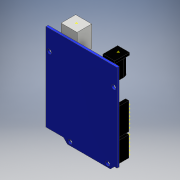
# Autodesk Inventor part: ArduinoUno
Saved by Autodesk Inventor 2016 (Build 200138000, 138)
## iProperties
Created: 2015-09-20
Part Number: ArduinoUno
Material: GFRP
Document SubType Name: Modeling
Designer: Artur
Density: 1.75 g/cm^3
Appearance: Smooth - Light Gray
Mass: 16.8005 g
Surface Area: 132.112 cm^2
Volume: 9.60028 cm^3
Author: Artur
Autodesk Inventor part; units mm, degrees
(part 1 of 3)
ref_plane "YZ Plane" through (0, 0, 0) normal (1, 0, 0) x (0, 1, 0)
ref_plane "XZ Plane" through (0, 0, 0) normal (0, 1, 0) x (-1, 0, 0)
sketch "Sketch1" plane through (0, 0, 0) normal (0, 1, 0) x (-1, 0, 0)
  line L0 (0, 0) -> (-53, 0)
  line L1 (-53, 0) -> (-53, -65)
  line L2 (-53, -65) -> (-51, -65)
  line L3 (-48, -68) -> (-16, -68)
  line L4 (-48, -68) -> (-51, -65)
  line L5 (0, -65) -> (-13, -65)
  circle A0 centre (-2.5, -15) radius 1.6
  circle A1 centre (-50.5, -13.9) radius 1.6
  circle A2 centre (-46, -65.5) radius 1.6
  circle A3 centre (-18, -65.5) radius 1.6
  line L6 (0, 0) -> (0, -93.7538) construction
  line L7 (-16, -68) -> (-13, -65)
  line L8 (0, -65) -> (0, 0)
  dimension "d0" = 53
  dimension "d1" = 65
  dimension "d2" = 2
  dimension "d3" = 32
  dimension "d4" = 68
  dimension "d5" = 5
  dimension "d6" = 13
  dimension "d7" = 3.2
  dimension "d9" = 15
  dimension "d10" = 3.2
  dimension "d11" = 1.1
  dimension "d12" = 2.5
  dimension "d13" = 3.2
  dimension "d14" = 3.2
  dimension "d15" = 7
  dimension "d16" = 65.5
  dimension "d17" = 35
  dimension "d18" = 65.5
  dimension "d20" = 2.5
  constraints: 18 end point, 4 centre point, 4 horizontal, 1 coincident, 1 collinear, 1 perpendicular, 1 point on line, 1 vertical
  measures "d0" distance of L0.start L0.end
  measures "d1" distance of L0.end L1.end
  measures "d2" distance of L1.end L2.end
  measures "d3" distance of L3.start L3.end
  measures "d4" distance between parallel lines of L0 L3
  measures "d5" distance from line of L1 L3.start
  measures "d6" distance of L5.start L5.end
  measures "d7" diameter of A0
  measures "d9" distance from line of L0 A0.centre
  measures "d10" diameter of A1
  measures "d11" vertical distance of A0.centre A1.centre
  measures "d12" distance from line of L1 A1.centre
  measures "d13" diameter of A2
  measures "d14" diameter of A3
  measures "d15" distance from line of L1 A2.centre
  measures "d16" distance from line of L0 A2.centre
  measures "d17" distance from line of L1 A3.centre
  measures "d18" distance from line of L0 A3.centre
  measures "d20" distance from line of L8 A0.centre
extrude "board" add sketch "Sketch1" against normal blind 1.6
sketch "Sketch2" plane through (0, 0, 0) normal (0, 1, 0) x (1, 0, 0)
  line L0 (9.6, 9.8) -> (9.6, -6.2)
  line L1 (9.6, -6.2) -> (21.6, -6.2)
  line L2 (21.6, -6.2) -> (21.6, 9.8)
  line L3 (21.6, 9.8) -> (9.6, 9.8)
  line L4 (0, 65) -> (0, 0) projected
  line L5 (0, 0) -> (53, 0) projected
  dimension "d23" = 16
  dimension "d24" = 12
  dimension "d25" = 9.6
  dimension "d26" = 9.8
  constraints: 8 end point, 3 perpendicular, 1 vertical
  measures "d23" distance of L0.start L0.end
  measures "d24" distance of L0.end L1.end
  measures "d25" distance between parallel lines of L4 L0
  measures "d26" distance between parallel lines of L5 L3
extrude "serialPort" add sketch "Sketch2" along normal blind 10.9 separate body
sketch "Sketch3" plane through (0, 0, 0) normal (0, 1, 0) x (1, 0, 0)
  line L0 (40.8, 12.2) -> (40.8, -1.8)
  line L1 (40.8, -1.8) -> (49.7, -1.8)
  line L2 (49.7, -1.8) -> (49.7, 12.2)
  line L3 (49.7, 12.2) -> (40.8, 12.2)
  line L4 (0, 0) -> (53, 0) projected
  line L5 (53, 0) -> (53, 65) projected
  dimension "d29" = 14
  dimension "d30" = 8.9
  dimension "d31" = 1.8
  dimension "d32" = 3.3
  constraints: 8 end point, 3 perpendicular, 1 vertical
  measures "d29" distance of L0.start L0.end
  measures "d30" distance of L0.end L1.end
  measures "d31" distance between parallel lines of L1 L4
  measures "d32" distance between parallel lines of L5 L2
extrude "powerPort" add sketch "Sketch3" along normal blind 11 separate body
sketch "Sketch4" plane through (0, 11, 0) normal (0, 1, 0) x (1, 0, 0)
  line L0 (0, 0) -> (53, 0) projected
split body "powerPortSplit" sketch "Sketch4" result two bodies bodies 3 curves L0 first body at (49.2, 3.6667, -4.0667)
fillet "powerPortFillet" radius 4.45 2 edges at (40.8, 11, -6.1) (49.7, 11, -6.1)
sketch "Sketch5" plane through (0, 0, 0) normal (0, 1, 0) x (1, 0, 0)
  line L0 (1.25, 43.5) -> (3.75, 43.5)
  line L1 (3.75, 43.5) -> (3.75, 18.5)
  line L2 (3.75, 18.5) -> (1.25, 18.5)
  line L3 (1.25, 18.5) -> (1.25, 43.5)
  line L4 (0, 65) -> (0, 0) projected
  line L5 (0, 0) -> (53, 0) projected
  line L6 (1.25, 64) -> (3.75, 64)
  line L7 (3.75, 64) -> (3.75, 44)
  line L8 (3.75, 44) -> (1.25, 44)
  line L9 (1.25, 44) -> (1.25, 64)
  line L10 (13, 65) -> (0, 65) projected
  line L11 (51.75, 64) -> (49.25, 64)
  line L12 (49.25, 64) -> (49.25, 49)
  line L13 (49.25, 49) -> (51.75, 49)
  line L14 (51.75, 49) -> (51.75, 64)
  line L15 (51.75, 47) -> (49.25, 47)
  line L16 (49.25, 27) -> (51.75, 27)
  line L17 (51.75, 47) -> (51.75, 27)
  line L18 (49.25, 47) -> (49.25, 27)
  point P0 (53, 65)
  dimension "d36" = 2.5
  dimension "d37" = 25
  dimension "d38" = 1.25
  dimension "d39" = 43.5
  dimension "d40" = 20
  dimension "d41" = 2.5
  dimension "d42" = 1
  dimension "d43" = 1.25
  dimension "d44" = 2.5
  dimension "d45" = 2.5
  dimension "d46" = 20
  dimension "d47" = 15
  dimension "d48" = 1.25
  dimension "d49" = 1
  dimension "d50" = 2
  constraints: 32 end point, 7 parallel, 4 horizontal, 3 perpendicular, 2 vertical, 1 point on line
  measures "d36" distance of L1.end L2.end
  measures "d37" distance of L0.end L1.end
  measures "d38" distance between parallel lines of L4 L3
  measures "d39" distance between parallel lines of L5 L0
  measures "d40" distance of L6.end L7.end
  measures "d41" distance of L7.end L8.end
  measures "d42" distance from line of L10 L6.start
  measures "d43" distance between parallel lines of L4 L9
  measures "d44" distance of L11.start L11.end
  measures "d45" distance of L15.start L15.end
  measures "d46" distance of L16.end L15.start
  measures "d47" distance of L13.end L11.start
  measures "d48" horizontal distance of point (53, 65) L11.start
  measures "d49" vertical distance of L11.start point (53, 65)
  measures "d50" distance of L15.start L13.end
extrude "pinsBase" add sketch "Sketch5" along normal blind 8.5 separate body
sketch "sketch6" plane through (0, 8.5, 0) normal (0, 1, 0) x (1, 0, 0)
  line L0 (1.5, 63.75) -> (3.5, 63.75)
  line L1 (3.5, 63.75) -> (3.5, 61.75)
  line L2 (3.5, 61.75) -> (1.5, 61.75)
  line L3 (1.5, 61.75) -> (1.5, 63.75)
  line L4 (3.75, 64) -> (1.25, 64) construction
  line L5 (1.25, 64) -> (1.25, 44) construction
  line L6 (1.5, 61.25) -> (3.5, 61.25)
  line L7 (3.5, 61.25) -> (3.5, 59.25)
  line L8 (3.5, 59.25) -> (1.5, 59.25)
  line L9 (1.5, 59.25) -> (1.5, 61.25)
  line L10 (1.5, 58.75) -> (3.5, 58.75)
  line L11 (3.5, 58.75) -> (3.5, 56.75)
  line L12 (3.5, 56.75) -> (1.5, 56.75)
  line L13 (1.5, 56.75) -> (1.5, 58.75)
  line L14 (1.5, 56.25) -> (3.5, 56.25)
  line L15 (3.5, 56.25) -> (3.5, 54.25)
  line L16 (3.5, 54.25) -> (1.5, 54.25)
  line L17 (1.5, 54.25) -> (1.5, 56.25)
  line L18 (1.5, 53.75) -> (3.5, 53.75)
  line L19 (3.5, 53.75) -> (3.5, 51.75)
  line L20 (3.5, 51.75) -> (1.5, 51.75)
  line L21 (1.5, 51.75) -> (1.5, 53.75)
  line L22 (1.5, 51.25) -> (3.5, 51.25)
  line L23 (3.5, 51.25) -> (3.5, 49.25)
  line L24 (3.5, 49.25) -> (1.5, 49.25)
  line L25 (1.5, 49.25) -> (1.5, 51.25)
  line L26 (1.5, 48.75) -> (3.5, 48.75)
  line L27 (3.5, 48.75) -> (3.5, 46.75)
  line L28 (3.5, 46.75) -> (1.5, 46.75)
  line L29 (1.5, 46.75) -> (1.5, 48.75)
  line L30 (1.5, 46.25) -> (3.5, 46.25)
  line L31 (3.5, 46.25) -> (3.5, 44.25)
  line L32 (3.5, 44.25) -> (1.5, 44.25)
  line L33 (1.5, 44.25) -> (1.5, 46.25)
  line L34 (3.75, 43.5) -> (1.25, 43.5) construction
  line L35 (1.25, 43.5) -> (1.25, 18.5) construction
  line L36 (1.5, 43.25) -> (3.5, 43.25)
  line L37 (3.5, 43.25) -> (3.5, 41.25)
  line L38 (3.5, 41.25) -> (1.5, 41.25)
  line L39 (1.5, 41.25) -> (1.5, 43.25)
  line L40 (1.5, 40.75) -> (3.5, 40.75)
  line L41 (3.5, 40.75) -> (3.5, 38.75)
  line L42 (3.5, 38.75) -> (1.5, 38.75)
  line L43 (1.5, 38.75) -> (1.5, 40.75)
  line L44 (1.5, 38.25) -> (3.5, 38.25)
  line L45 (3.5, 38.25) -> (3.5, 36.25)
  line L46 (3.5, 36.25) -> (1.5, 36.25)
  line L47 (1.5, 36.25) -> (1.5, 38.25)
  line L48 (1.5, 35.75) -> (3.5, 35.75)
  line L49 (3.5, 35.75) -> (3.5, 33.75)
  line L50 (3.5, 33.75) -> (1.5, 33.75)
  line L51 (1.5, 33.75) -> (1.5, 35.75)
  line L52 (1.5, 33.25) -> (3.5, 33.25)
  line L53 (3.5, 33.25) -> (3.5, 31.25)
  line L54 (3.5, 31.25) -> (1.5, 31.25)
  line L55 (1.5, 31.25) -> (1.5, 33.25)
  line L56 (1.5, 30.75) -> (3.5, 30.75)
  line L57 (3.5, 30.75) -> (3.5, 28.75)
  line L58 (3.5, 28.75) -> (1.5, 28.75)
  line L59 (1.5, 28.75) -> (1.5, 30.75)
  line L60 (1.5, 28.25) -> (3.5, 28.25)
  line L61 (3.5, 28.25) -> (3.5, 26.25)
  line L62 (3.5, 26.25) -> (1.5, 26.25)
  line L63 (1.5, 26.25) -> (1.5, 28.25)
  line L64 (1.5, 25.75) -> (3.5, 25.75)
  line L65 (3.5, 25.75) -> (3.5, 23.75)
  line L66 (3.5, 23.75) -> (1.5, 23.75)
  line L67 (1.5, 23.75) -> (1.5, 25.75)
  line L68 (1.5, 23.25) -> (3.5, 23.25)
  line L69 (3.5, 23.25) -> (3.5, 21.25)
  line L70 (3.5, 21.25) -> (1.5, 21.25)
  line L71 (1.5, 21.25) -> (1.5, 23.25)
  line L72 (1.5, 20.75) -> (3.5, 20.75)
  line L73 (3.5, 20.75) -> (3.5, 18.75)
  line L74 (3.5, 18.75) -> (1.5, 18.75)
  line L75 (1.5, 18.75) -> (1.5, 20.75)
  line L76 (49.5, 63.75) -> (51.5, 63.75)
  line L77 (51.5, 63.75) -> (51.5, 61.75)
  line L78 (51.5, 61.75) -> (49.5, 61.75)
  line L79 (49.5, 61.75) -> (49.5, 63.75)
  line L80 (49.5, 46.75) -> (51.5, 46.75)
  line L81 (51.5, 46.75) -> (51.5, 44.75)
  line L82 (51.5, 44.75) -> (49.5, 44.75)
  line L83 (49.5, 44.75) -> (49.5, 46.75)
  line L84 (51.75, 64) -> (49.25, 64) construction
  line L85 (49.25, 64) -> (49.25, 49) construction
  line L86 (51.75, 47) -> (49.25, 47) construction
  line L87 (49.25, 47) -> (49.25, 27) construction
  line L88 (51.5, 59.25) -> (49.5, 59.25)
  line L89 (49.5, 59.25) -> (49.5, 61.25)
  line L90 (49.5, 61.25) -> (51.5, 61.25)
  line L91 (51.5, 61.25) -> (51.5, 59.25)
  line L92 (51.5, 56.75) -> (49.5, 56.75)
  line L93 (49.5, 56.75) -> (49.5, 58.75)
  line L94 (49.5, 58.75) -> (51.5, 58.75)
  line L95 (51.5, 58.75) -> (51.5, 56.75)
  line L96 (51.5, 54.25) -> (49.5, 54.25)
  line L97 (49.5, 54.25) -> (49.5, 56.25)
  line L98 (49.5, 56.25) -> (51.5, 56.25)
  line L99 (51.5, 56.25) -> (51.5, 54.25)
  line L100 (51.5, 51.75) -> (49.5, 51.75)
  line L101 (49.5, 51.75) -> (49.5, 53.75)
  line L102 (49.5, 53.75) -> (51.5, 53.75)
  line L103 (51.5, 53.75) -> (51.5, 51.75)
  line L104 (51.5, 49.25) -> (49.5, 49.25)
  line L105 (49.5, 49.25) -> (49.5, 51.25)
  line L106 (49.5, 51.25) -> (51.5, 51.25)
  line L107 (51.5, 51.25) -> (51.5, 49.25)
  line L108 (49.5, 44.25) -> (51.5, 44.25)
  line L109 (49.5, 42.25) -> (49.5, 44.25)
  line L110 (51.5, 42.25) -> (49.5, 42.25)
  line L111 (51.5, 44.25) -> (51.5, 42.25)
  line L112 (49.5, 41.75) -> (51.5, 41.75)
  line L113 (49.5, 39.75) -> (49.5, 41.75)
  line L114 (51.5, 39.75) -> (49.5, 39.75)
  line L115 (51.5, 41.75) -> (51.5, 39.75)
  line L116 (49.5, 39.25) -> (51.5, 39.25)
  line L117 (49.5, 37.25) -> (49.5, 39.25)
  line L118 (51.5, 37.25) -> (49.5, 37.25)
  line L119 (51.5, 39.25) -> (51.5, 37.25)
  line L120 (49.5, 36.75) -> (51.5, 36.75)
  line L121 (49.5, 34.75) -> (49.5, 36.75)
  line L122 (51.5, 34.75) -> (49.5, 34.75)
  line L123 (51.5, 36.75) -> (51.5, 34.75)
  line L124 (49.5, 34.25) -> (51.5, 34.25)
  line L125 (49.5, 32.25) -> (49.5, 34.25)
  line L126 (51.5, 32.25) -> (49.5, 32.25)
  line L127 (51.5, 34.25) -> (51.5, 32.25)
  line L128 (49.5, 31.75) -> (51.5, 31.75)
  line L129 (49.5, 29.75) -> (49.5, 31.75)
  line L130 (51.5, 29.75) -> (49.5, 29.75)
  line L131 (51.5, 31.75) -> (51.5, 29.75)
  line L132 (49.5, 29.25) -> (51.5, 29.25)
  line L133 (49.5, 27.25) -> (49.5, 29.25)
  line L134 (51.5, 27.25) -> (49.5, 27.25)
  line L135 (51.5, 29.25) -> (51.5, 27.25)
  point P0 (0, 0)
  dimension "d53" = 2
  dimension "d54" = 2
  dimension "d55" = 0.25
  dimension "d56" = 0.25
  dimension "d61" = 2.5
  dimension "d70" = 2
  dimension "d71" = 2
  dimension "d72" = 0.25
  dimension "d73" = 0.25
  dimension "d76" = 2.5
  dimension "d89" = 2
  dimension "d90" = 2
  dimension "d99" = 2
  dimension "d100" = 2
  dimension "d101" = 0.25
  dimension "d102" = 0.25
  dimension "d103" = 0.25
  dimension "d104" = 0.25
  dimension "d107" = 2.5
  dimension "d114" = 2.5
  constraints: 256 end point, 8 parallel, 4 horizontal, 4 perpendicular, 4 vertical, 224 other
  measures "d53" distance of L1.end L2.end
  measures "d54" distance of L0.end L1.end
  measures "d55" distance from line of L4 L0.end
  measures "d56" distance from line of L5 L0.start
  measures "d61" distance of L0.start L6.start
  measures "d70" distance of L37.end L38.end
  measures "d71" distance of L37.start L37.end
  measures "d72" distance between parallel lines of L34 L36
  measures "d73" distance between parallel lines of L35 L39
  measures "d76" distance of L37.start L40.end
  measures "d89" distance of L78.start L78.end
  measures "d90" distance of L76.end L78.start
  measures "d99" distance of L82.start L82.end
  measures "d100" distance of L80.end L82.start
  measures "d101" distance between parallel lines of L86 L80
  measures "d102" distance between parallel lines of L87 L83
  measures "d103" distance between parallel lines of L84 L76
  measures "d104" distance between parallel lines of L85 L79
  measures "d107" distance of L78.end L88.end
  measures "d114" distance of L80.end L108.end
extrude "pinHoles" cut sketch "sketch6" against normal up to next bodies 6
sketch "pinLabelsSketch" plane through (0, 0, 0) normal (0, 1, 0) x (1, 0, 0)
  line L0 (10.8569, 44) -> (4, 44) construction
  line L1 (4, 44) -> (4, 64) construction
  line L2 (4, 64) -> (10.8569, 64) construction
  line L3 (10.8569, 64) -> (10.8569, 44) construction
  line L4 (3.5, 61.75) -> (1.5, 61.75) construction
  line L5 (3.75, 44) -> (3.75, 64) construction
  line L6 (1.25, 44) -> (3.75, 44) construction
  line L7 (3.75, 64) -> (1.25, 64) construction
  line L8 (10.2543, 23.75) -> (4, 23.75) construction
  line L9 (4, 23.75) -> (4, 43.5) construction
  line L10 (4, 43.5) -> (10.2543, 43.5) construction
  line L11 (10.2543, 43.5) -> (10.2543, 23.75) construction
  line L12 (3.75, 18.5) -> (3.75, 43.5) construction
  line L13 (1.25, 18.5) -> (3.75, 18.5) construction
  line L14 (3.75, 43.5) -> (1.25, 43.5) construction
  line L15 (3.5, 23.75) -> (1.5, 23.75) construction
  line L16 (49, 49) -> (44.6855, 49) construction
  line L17 (44.6855, 49) -> (44.6855, 64) construction
  line L18 (44.6855, 64) -> (49, 64) construction
  line L19 (49, 64) -> (49, 49) construction
  line L20 (49.25, 64) -> (49.25, 49) construction
  line L21 (51.75, 64) -> (49.25, 64) construction
  line L22 (49.25, 49) -> (51.75, 49) projected
  line L23 (49, 47) -> (49, 29.75) construction
  line L24 (49, 29.75) -> (42.6731, 29.75) construction
  line L25 (42.6731, 29.75) -> (42.6731, 47) construction
  line L26 (42.6731, 47) -> (49, 47) construction
  line L27 (49.25, 47) -> (49.25, 27) construction
  line L28 (49.25, 27) -> (51.75, 27) projected
  line L29 (51.75, 47) -> (49.25, 47) construction
  line L30 (51.5, 29.75) -> (49.5, 29.75) construction
  line L31 (48.3254, 31.6408) -> (48.9064, 31.6408)
  line L32 (48.9064, 31.6408) -> (48.9064, 31.4876)
  line L33 (48.9064, 31.4876) -> (48.7156, 31.4876)
  line L34 (48.7156, 31.4876) -> (48.7156, 30.294)
  line L35 (48.7156, 30.294) -> (48.9064, 30.294)
  line L36 (48.9064, 30.294) -> (48.9064, 30.1408)
  line L37 (48.9064, 30.1408) -> (48.3254, 30.1408)
  line L38 (48.3254, 30.1408) -> (48.3254, 30.294)
  line L39 (48.3254, 30.294) -> (48.5162, 30.294)
  line L40 (48.5162, 30.294) -> (48.5162, 31.4876)
  line L41 (48.5162, 31.4876) -> (48.3254, 31.4876)
  line L42 (48.3254, 31.4876) -> (48.3254, 31.6408)
  spline S0 degree 2 poles (47.0174, 30.3122) (46.9323, 30.4119) (46.8375, 30.7036) (46.8375, 30.8908) knots 0 0 0 1 2 2 2
  spline S1 degree 2 poles (46.8375, 30.8908) (46.8375, 31.0731) (46.9299, 31.3685) (47.0174, 31.4682) knots 0 0 0 1 2 2 2
  spline S2 degree 2 poles (47.0174, 31.4682) (47.1098, 31.5727) (47.3541, 31.6724) (47.5012, 31.6724) knots 0 0 0 1 2 2 2
  spline S3 degree 2 poles (47.5012, 31.6724) (47.6532, 31.6724) (47.8963, 31.5691) (47.985, 31.4682) knots 0 0 0 1 2 2 2
  spline S4 degree 2 poles (47.985, 31.4682) (48.0713, 31.3685) (48.1637, 31.0756) (48.1637, 30.8908) knots 0 0 0 1 2 2 2
  spline S5 degree 2 poles (48.1637, 30.8908) (48.1637, 30.7024) (48.0701, 30.4155) (47.9838, 30.3122) knots 0 0 0 1 2 2 2
  spline S6 degree 2 poles (47.9838, 30.3122) (47.8963, 30.2125) (47.6519, 30.1092) (47.5012, 30.1092) knots 0 0 0 1 2 2 2
  spline S7 degree 2 poles (47.5012, 30.1092) (47.3481, 30.1092) (47.1025, 30.2162) (47.0174, 30.3122) knots 0 0 0 1 2 2 2
  spline S8 degree 2 poles (47.0454, 30.8908) (47.0454, 30.7425) (47.1098, 30.5128) (47.1682, 30.4374) knots 0 0 0 1 2 2 2
  spline S9 degree 2 poles (47.1682, 30.4374) (47.2277, 30.3596) (47.3955, 30.2818) (47.5, 30.2818) knots 0 0 0 1 2 2 2
  spline S10 degree 2 poles (47.5, 30.2818) (47.6082, 30.2818) (47.7711, 30.3572) (47.8331, 30.4374) knots 0 0 0 1 2 2 2
  spline S11 degree 2 poles (47.8331, 30.4374) (47.8926, 30.514) (47.9558, 30.7449) (47.9558, 30.8908) knots 0 0 0 1 2 2 2
  spline S12 degree 2 poles (47.9558, 30.8908) (47.9558, 31.1862) (47.7079, 31.4998) (47.5, 31.4998) knots 0 0 0 1 2 2 2
  spline S13 degree 2 poles (47.5, 31.4998) (47.2921, 31.4998) (47.0454, 31.1862) (47.0454, 30.8908) knots 0 0 0 1 2 2 2
  line L43 (45.4579, 31.6408) -> (45.7168, 31.6408)
  line L44 (45.7168, 31.6408) -> (46.1908, 31.044)
  line L45 (46.1908, 31.044) -> (46.4194, 31.044)
  line L46 (46.4194, 31.044) -> (46.4194, 31.6408)
  line L47 (46.4194, 31.6408) -> (46.6187, 31.6408)
  line L48 (46.6187, 31.6408) -> (46.6187, 30.1408)
  line L49 (46.6187, 30.1408) -> (46.2322, 30.1408)
  spline S14 degree 2 poles (46.2322, 30.1408) (46.1033, 30.1408) (45.9295, 30.1688) (45.8505, 30.2198) knots 0 0 0 1 2 2 2
  spline S15 degree 2 poles (45.8505, 30.2198) (45.7715, 30.2709) (45.6803, 30.4301) (45.6803, 30.548) knots 0 0 0 1 2 2 2
  spline S16 degree 2 poles (45.6803, 30.548) (45.6803, 30.7121) (45.8481, 30.9346) (45.9915, 30.988) knots 0 0 0 1 2 2 2
  line L50 (45.9915, 30.988) -> (45.4579, 31.6408)
  spline S17 degree 2 poles (45.8882, 30.5638) (45.8882, 30.4982) (45.9344, 30.3973) (45.983, 30.3645) knots 0 0 0 1 2 2 2
  spline S18 degree 2 poles (45.983, 30.3645) (46.0255, 30.3365) (46.1386, 30.3134) (46.2212, 30.3134) knots 0 0 0 1 2 2 2
  line L51 (46.2212, 30.3134) -> (46.4194, 30.3134)
  line L52 (46.4194, 30.3134) -> (46.4194, 30.8774)
  line L53 (46.4194, 30.8774) -> (46.2443, 30.8774)
  spline S19 degree 2 poles (46.2443, 30.8774) (46.158, 30.8774) (46.0207, 30.847) (45.9733, 30.7996) knots 0 0 0 1 2 2 2
  spline S20 degree 2 poles (45.9733, 30.7996) (45.9295, 30.7583) (45.8882, 30.6416) (45.8882, 30.5638) knots 0 0 0 1 2 2 2
  line L54 (45.3387, 31.6408) -> (45.3387, 30.1408)
  line L55 (45.3387, 30.1408) -> (44.4003, 30.1408)
  line L56 (44.4003, 30.1408) -> (44.4003, 30.3183)
  line L57 (44.4003, 30.3183) -> (45.1394, 30.3183)
  line L58 (45.1394, 30.3183) -> (45.1394, 30.7291)
  line L59 (45.1394, 30.7291) -> (44.4502, 30.7291)
  line L60 (44.4502, 30.7291) -> (44.4502, 30.9066)
  line L61 (44.4502, 30.9066) -> (45.1394, 30.9066)
  line L62 (45.1394, 30.9066) -> (45.1394, 31.4633)
  line L63 (45.1394, 31.4633) -> (44.4003, 31.4633)
  line L64 (44.4003, 31.4633) -> (44.4003, 31.6408)
  line L65 (44.4003, 31.6408) -> (45.3387, 31.6408)
  line L66 (43.2844, 30.3183) -> (43.9822, 30.3183)
  line L67 (43.9822, 30.3183) -> (43.9822, 30.7413)
  line L68 (43.9822, 30.7413) -> (43.3136, 30.7413)
  line L69 (43.3136, 30.7413) -> (43.3136, 30.9188)
  line L70 (43.3136, 30.9188) -> (43.9822, 30.9188)
  line L71 (43.9822, 30.9188) -> (43.9822, 31.6408)
  line L72 (43.9822, 31.6408) -> (44.1815, 31.6408)
  line L73 (44.1815, 31.6408) -> (44.1815, 30.1408)
  line L74 (44.1815, 30.1408) -> (43.2844, 30.1408)
  line L75 (43.2844, 30.1408) -> (43.2844, 30.3183)
  line L76 (47.6872, 34.1408) -> (47.9461, 34.1408)
  line L77 (47.9461, 34.1408) -> (48.4202, 33.544)
  line L78 (48.4202, 33.544) -> (48.6487, 33.544)
  line L79 (48.6487, 33.544) -> (48.6487, 34.1408)
  line L80 (48.6487, 34.1408) -> (48.8481, 34.1408)
  line L81 (48.8481, 34.1408) -> (48.8481, 32.6408)
  line L82 (48.8481, 32.6408) -> (48.4615, 32.6408)
  spline S21 degree 2 poles (48.4615, 32.6408) (48.3327, 32.6408) (48.1588, 32.6688) (48.0798, 32.7198) knots 0 0 0 1 2 2 2
  spline S22 degree 2 poles (48.0798, 32.7198) (48.0008, 32.7709) (47.9096, 32.9301) (47.9096, 33.048) knots 0 0 0 1 2 2 2
  spline S23 degree 2 poles (47.9096, 33.048) (47.9096, 33.2121) (48.0774, 33.4346) (48.2208, 33.488) knots 0 0 0 1 2 2 2
  line L83 (48.2208, 33.488) -> (47.6872, 34.1408)
  spline S24 degree 2 poles (48.1175, 33.0638) (48.1175, 32.9982) (48.1637, 32.8973) (48.2123, 32.8645) knots 0 0 0 1 2 2 2
  spline S25 degree 2 poles (48.2123, 32.8645) (48.2549, 32.8365) (48.3679, 32.8134) (48.4506, 32.8134) knots 0 0 0 1 2 2 2
  line L84 (48.4506, 32.8134) -> (48.6487, 32.8134)
  line L85 (48.6487, 32.8134) -> (48.6487, 33.3774)
  line L86 (48.6487, 33.3774) -> (48.4737, 33.3774)
  spline S26 degree 2 poles (48.4737, 33.3774) (48.3874, 33.3774) (48.25, 33.347) (48.2026, 33.2996) knots 0 0 0 1 2 2 2
  spline S27 degree 2 poles (48.2026, 33.2996) (48.1588, 33.2583) (48.1175, 33.1416) (48.1175, 33.0638) knots 0 0 0 1 2 2 2
  line L87 (47.5681, 34.1408) -> (47.5681, 32.6408)
  line L88 (47.5681, 32.6408) -> (46.6297, 32.6408)
  line L89 (46.6297, 32.6408) -> (46.6297, 32.8183)
  line L90 (46.6297, 32.8183) -> (47.3687, 32.8183)
  line L91 (47.3687, 32.8183) -> (47.3687, 33.2291)
  line L92 (47.3687, 33.2291) -> (46.6795, 33.2291)
  line L93 (46.6795, 33.2291) -> (46.6795, 33.4066)
  line L94 (46.6795, 33.4066) -> (47.3687, 33.4066)
  line L95 (47.3687, 33.4066) -> (47.3687, 33.9633)
  line L96 (47.3687, 33.9633) -> (46.6297, 33.9633)
  line L97 (46.6297, 33.9633) -> (46.6297, 34.1408)
  line L98 (46.6297, 34.1408) -> (47.5681, 34.1408)
  spline S28 degree 2 poles (45.9927, 34.1675) (46.1556, 34.1675) (46.3841, 34.0995) (46.485, 34.0509) knots 0 0 0 1 2 2 2
  line L99 (46.485, 34.0509) -> (46.485, 33.8004)
  line L100 (46.485, 33.8004) -> (46.4704, 33.8004)
  spline S29 degree 2 poles (46.4704, 33.8004) (46.372, 33.8928) (46.1228, 33.9949) (46.0073, 33.9949) knots 0 0 0 1 2 2 2
  spline S30 degree 2 poles (46.0073, 33.9949) (45.842, 33.9949) (45.673, 33.8576) (45.673, 33.7445) knots 0 0 0 1 2 2 2
  spline S31 degree 2 poles (45.673, 33.7445) (45.673, 33.6546) (45.7618, 33.5427) (45.8578, 33.5148) knots 0 0 0 1 2 2 2
  spline S32 degree 2 poles (45.8578, 33.5148) (45.9271, 33.4953) (46.0425, 33.4686) (46.1288, 33.4467) knots 0 0 0 1 2 2 2
  spline S33 degree 2 poles (46.1288, 33.4467) (46.2066, 33.4261) (46.3294, 33.3641) (46.3768, 33.3142) knots 0 0 0 1 2 2 2
  spline S34 degree 2 poles (46.3768, 33.3142) (46.423, 33.2644) (46.4741, 33.1307) (46.4741, 33.0432) knots 0 0 0 1 2 2 2
  spline S35 degree 2 poles (46.4741, 33.0432) (46.4741, 32.8608) (46.1896, 32.6141) (45.9696, 32.6141) knots 0 0 0 1 2 2 2
  spline S36 degree 2 poles (45.9696, 32.6141) (45.8432, 32.6141) (45.6195, 32.6639) (45.5235, 32.7113) knots 0 0 0 1 2 2 2
  line L101 (45.5235, 32.7113) -> (45.5235, 32.9496)
  line L102 (45.5235, 32.9496) -> (45.5381, 32.9496)
  spline S37 degree 2 poles (45.5381, 32.9496) (45.6098, 32.8839) (45.8335, 32.7867) (45.9562, 32.7867) knots 0 0 0 1 2 2 2
  spline S38 degree 2 poles (45.9562, 32.7867) (46.0948, 32.7867) (46.2662, 32.9167) (46.2662, 33.0225) knots 0 0 0 1 2 2 2
  spline S39 degree 2 poles (46.2662, 33.0225) (46.2662, 33.1173) (46.1653, 33.2303) (46.0705, 33.2559) knots 0 0 0 1 2 2 2
  spline S40 degree 2 poles (46.0705, 33.2559) (46.0073, 33.2729) (45.8237, 33.3167) (45.763, 33.3349) knots 0 0 0 1 2 2 2
  spline S41 degree 2 poles (45.763, 33.3349) (45.6086, 33.3823) (45.4652, 33.5731) (45.4652, 33.7129) knots 0 0 0 1 2 2 2
  spline S42 degree 2 poles (45.4652, 33.7129) (45.4652, 33.8017) (45.5369, 33.9718) (45.6013, 34.0314) knots 0 0 0 1 2 2 2
  spline S43 degree 2 poles (45.6013, 34.0314) (45.673, 34.097) (45.8553, 34.1675) (45.9927, 34.1675) knots 0 0 0 1 2 2 2
  line L103 (45.2622, 34.1408) -> (45.2622, 32.6408)
  line L104 (45.2622, 32.6408) -> (44.3237, 32.6408)
  line L105 (44.3237, 32.6408) -> (44.3237, 32.8183)
  line L106 (44.3237, 32.8183) -> (45.0628, 32.8183)
  line L107 (45.0628, 32.8183) -> (45.0628, 33.2291)
  line L108 (45.0628, 33.2291) -> (44.3736, 33.2291)
  line L109 (44.3736, 33.2291) -> (44.3736, 33.4066)
  line L110 (44.3736, 33.4066) -> (45.0628, 33.4066)
  line L111 (45.0628, 33.4066) -> (45.0628, 33.9633)
  line L112 (45.0628, 33.9633) -> (44.3237, 33.9633)
  line L113 (44.3237, 33.9633) -> (44.3237, 34.1408)
  line L114 (44.3237, 34.1408) -> (45.2622, 34.1408)
  line L115 (43.7549, 34.1408) -> (43.7549, 32.8183)
  line L116 (43.7549, 32.8183) -> (44.2581, 32.8183)
  line L117 (44.2581, 32.8183) -> (44.2581, 32.6408)
  line L118 (44.2581, 32.6408) -> (43.0523, 32.6408)
  line L119 (43.0523, 32.6408) -> (43.0523, 32.8183)
  line L120 (43.0523, 32.8183) -> (43.5555, 32.8183)
  line L121 (43.5555, 32.8183) -> (43.5555, 34.1408)
  line L122 (43.5555, 34.1408) -> (43.7549, 34.1408)
  spline S44 degree 2 poles (48.4858, 35.283) (48.5405, 35.283) (48.6487, 35.3098) (48.701, 35.3304) knots 0 0 0 1 2 2 2
  spline S45 degree 2 poles (48.701, 35.3304) (48.7496, 35.3511) (48.8213, 35.3949) (48.8493, 35.4143) knots 0 0 0 1 2 2 2
  line L123 (48.8493, 35.4143) -> (48.8614, 35.4143)
  line L124 (48.8614, 35.4143) -> (48.8614, 35.2016)
  spline S46 degree 2 poles (48.8614, 35.2016) (48.7958, 35.1663) (48.5709, 35.1092) (48.47, 35.1092) knots 0 0 0 1 2 2 2
  spline S47 degree 2 poles (48.47, 35.1092) (48.3679, 35.1092) (48.216, 35.1505) (48.154, 35.1943) knots 0 0 0 1 2 2 2
  spline S48 degree 2 poles (48.154, 35.1943) (48.0883, 35.2417) (48.0203, 35.3791) (48.0203, 35.4714) knots 0 0 0 1 2 2 2
  spline S49 degree 2 poles (48.0203, 35.4714) (48.0203, 35.5954) (48.1831, 35.7826) (48.2974, 35.8069) knots 0 0 0 1 2 2 2
  line L125 (48.2974, 35.8069) -> (48.2974, 35.8215)
  spline S50 degree 2 poles (48.2974, 35.8215) (48.25, 35.8312) (48.1418, 35.875) (48.0956, 35.9188) knots 0 0 0 1 2 2 2
  spline S51 degree 2 poles (48.0956, 35.9188) (48.0494, 35.9613) (47.9911, 36.0974) (47.9911, 36.1959) knots 0 0 0 1 2 2 2
  spline S52 degree 2 poles (47.9911, 36.1959) (47.9911, 36.2968) (48.0604, 36.4682) (48.1236, 36.5338) knots 0 0 0 1 2 2 2
  spline S53 degree 2 poles (48.1236, 36.5338) (48.1892, 36.6019) (48.3752, 36.6724) (48.4931, 36.6724) knots 0 0 0 1 2 2 2
  spline S54 degree 2 poles (48.4931, 36.6724) (48.6062, 36.6724) (48.8274, 36.6177) (48.9028, 36.58) knots 0 0 0 1 2 2 2
  line L126 (48.9028, 36.58) -> (48.9028, 36.3673)
  line L127 (48.9028, 36.3673) -> (48.8882, 36.3673)
  spline S55 degree 2 poles (48.8882, 36.3673) (48.825, 36.4135) (48.611, 36.4986) (48.5053, 36.4986) knots 0 0 0 1 2 2 2
  spline S56 degree 2 poles (48.5053, 36.4986) (48.4433, 36.4986) (48.3193, 36.4597) (48.278, 36.4147) knots 0 0 0 1 2 2 2
  spline S57 degree 2 poles (48.278, 36.4147) (48.2378, 36.3697) (48.1953, 36.2628) (48.1953, 36.1813) knots 0 0 0 1 2 2 2
  spline S58 degree 2 poles (48.1953, 36.1813) (48.1953, 36.0999) (48.2427, 35.9941) (48.2853, 35.9637) knots 0 0 0 1 2 2 2
  spline S59 degree 2 poles (48.2853, 35.9637) (48.3278, 35.9333) (48.4433, 35.9103) (48.5113, 35.9103) knots 0 0 0 1 2 2 2
  line L128 (48.5113, 35.9103) -> (48.5964, 35.9103)
  line L129 (48.5964, 35.9103) -> (48.5964, 35.7437)
  line L130 (48.5964, 35.7437) -> (48.5296, 35.7437)
  spline S60 degree 2 poles (48.5296, 35.7437) (48.3947, 35.7437) (48.2245, 35.6149) (48.2245, 35.4921) knots 0 0 0 1 2 2 2
  spline S61 degree 2 poles (48.2245, 35.4921) (48.2245, 35.435) (48.2682, 35.3535) (48.3035, 35.3292) knots 0 0 0 1 2 2 2
  spline S62 degree 2 poles (48.3035, 35.3292) (48.3412, 35.3037) (48.4335, 35.283) (48.4858, 35.283) knots 0 0 0 1 2 2 2
  line L131 (47.4429, 36.6408) -> (47.6835, 36.6408)
  line L132 (47.6835, 36.6408) -> (47.6835, 36.3539)
  line L133 (47.6835, 36.3539) -> (47.4429, 36.3539)
  line L134 (47.4429, 36.3539) -> (47.4429, 36.6408)
  spline S63 degree 2 poles (46.7354, 35.283) (46.7901, 35.283) (46.8983, 35.3098) (46.9506, 35.3304) knots 0 0 0 1 2 2 2
  spline S64 degree 2 poles (46.9506, 35.3304) (46.9992, 35.3511) (47.0709, 35.3949) (47.0989, 35.4143) knots 0 0 0 1 2 2 2
  line L135 (47.0989, 35.4143) -> (47.111, 35.4143)
  line L136 (47.111, 35.4143) -> (47.111, 35.2016)
  spline S65 degree 2 poles (47.111, 35.2016) (47.0454, 35.1663) (46.8205, 35.1092) (46.7196, 35.1092) knots 0 0 0 1 2 2 2
  spline S66 degree 2 poles (46.7196, 35.1092) (46.6175, 35.1092) (46.4656, 35.1505) (46.4036, 35.1943) knots 0 0 0 1 2 2 2
  spline S67 degree 2 poles (46.4036, 35.1943) (46.3379, 35.2417) (46.2699, 35.3791) (46.2699, 35.4714) knots 0 0 0 1 2 2 2
  spline S68 degree 2 poles (46.2699, 35.4714) (46.2699, 35.5954) (46.4327, 35.7826) (46.547, 35.8069) knots 0 0 0 1 2 2 2
  line L137 (46.547, 35.8069) -> (46.547, 35.8215)
  spline S69 degree 2 poles (46.547, 35.8215) (46.4996, 35.8312) (46.3914, 35.875) (46.3452, 35.9188) knots 0 0 0 1 2 2 2
  spline S70 degree 2 poles (46.3452, 35.9188) (46.299, 35.9613) (46.2407, 36.0974) (46.2407, 36.1959) knots 0 0 0 1 2 2 2
  spline S71 degree 2 poles (46.2407, 36.1959) (46.2407, 36.2968) (46.31, 36.4682) (46.3732, 36.5338) knots 0 0 0 1 2 2 2
  spline S72 degree 2 poles (46.3732, 36.5338) (46.4388, 36.6019) (46.6248, 36.6724) (46.7427, 36.6724) knots 0 0 0 1 2 2 2
  spline S73 degree 2 poles (46.7427, 36.6724) (46.8558, 36.6724) (47.077, 36.6177) (47.1524, 36.58) knots 0 0 0 1 2 2 2
  line L138 (47.1524, 36.58) -> (47.1524, 36.3673)
  line L139 (47.1524, 36.3673) -> (47.1378, 36.3673)
  spline S74 degree 2 poles (47.1378, 36.3673) (47.0746, 36.4135) (46.8606, 36.4986) (46.7549, 36.4986) knots 0 0 0 1 2 2 2
  spline S75 degree 2 poles (46.7549, 36.4986) (46.6929, 36.4986) (46.5689, 36.4597) (46.5276, 36.4147) knots 0 0 0 1 2 2 2
  spline S76 degree 2 poles (46.5276, 36.4147) (46.4874, 36.3697) (46.4449, 36.2628) (46.4449, 36.1813) knots 0 0 0 1 2 2 2
  spline S77 degree 2 poles (46.4449, 36.1813) (46.4449, 36.0999) (46.4923, 35.9941) (46.5348, 35.9637) knots 0 0 0 1 2 2 2
  spline S78 degree 2 poles (46.5348, 35.9637) (46.5774, 35.9333) (46.6929, 35.9103) (46.7609, 35.9103) knots 0 0 0 1 2 2 2
  line L140 (46.7609, 35.9103) -> (46.846, 35.9103)
  line L141 (46.846, 35.9103) -> (46.846, 35.7437)
  line L142 (46.846, 35.7437) -> (46.7792, 35.7437)
  spline S79 degree 2 poles (46.7792, 35.7437) (46.6442, 35.7437) (46.4741, 35.6149) (46.4741, 35.4921) knots 0 0 0 1 2 2 2
  spline S80 degree 2 poles (46.4741, 35.4921) (46.4741, 35.435) (46.5178, 35.3535) (46.5531, 35.3292) knots 0 0 0 1 2 2 2
  spline S81 degree 2 poles (46.5531, 35.3292) (46.5908, 35.3037) (46.6831, 35.283) (46.7354, 35.283) knots 0 0 0 1 2 2 2
  line L143 (44.8841, 35.1408) -> (45.4007, 36.6408)
  line L144 (45.4007, 36.6408) -> (45.6159, 36.6408)
  line L145 (45.6159, 36.6408) -> (46.1325, 35.1408)
  line L146 (46.1325, 35.1408) -> (45.9186, 35.1408)
  line L147 (45.9186, 35.1408) -> (45.5028, 36.3868)
  line L148 (45.5028, 36.3868) -> (45.0871, 35.1408)
  line L149 (45.0871, 35.1408) -> (44.8841, 35.1408)
  spline S82 degree 2 poles (47.9814, 38.6643) (47.9814, 38.7725) (48.0506, 38.9573) (48.1139, 39.0253) knots 0 0 0 1 2 2 2
  spline S83 degree 2 poles (48.1139, 39.0253) (48.1771, 39.0934) (48.3655, 39.1724) (48.4822, 39.1724) knots 0 0 0 1 2 2 2
  spline S84 degree 2 poles (48.4822, 39.1724) (48.5891, 39.1724) (48.7982, 39.125) (48.8748, 39.0873) knots 0 0 0 1 2 2 2
  line L150 (48.8748, 39.0873) -> (48.8748, 38.8746)
  line L151 (48.8748, 38.8746) -> (48.8602, 38.8746)
  spline S85 degree 2 poles (48.8602, 38.8746) (48.8371, 38.8916) (48.7508, 38.9354) (48.6985, 38.9548) knots 0 0 0 1 2 2 2
  spline S86 degree 2 poles (48.6985, 38.9548) (48.639, 38.9755) (48.5405, 38.9986) (48.4785, 38.9986) knots 0 0 0 1 2 2 2
  spline S87 degree 2 poles (48.4785, 38.9986) (48.4177, 38.9986) (48.3035, 38.9548) (48.2622, 38.9074) knots 0 0 0 1 2 2 2
  spline S88 degree 2 poles (48.2622, 38.9074) (48.2245, 38.8624) (48.1856, 38.7433) (48.1856, 38.6631) knots 0 0 0 1 2 2 2
  spline S89 degree 2 poles (48.1856, 38.6631) (48.1856, 38.5829) (48.2293, 38.4808) (48.2707, 38.4467) knots 0 0 0 1 2 2 2
  spline S90 degree 2 poles (48.2707, 38.4467) (48.3132, 38.409) (48.4396, 38.3774) (48.5162, 38.3774) knots 0 0 0 1 2 2 2
  spline S91 degree 2 poles (48.5162, 38.3774) (48.5989, 38.3774) (48.763, 38.403) (48.8128, 38.4139) knots 0 0 0 1 2 2 2
  line L152 (48.8128, 38.4139) -> (48.8128, 37.6408)
  line L153 (48.8128, 37.6408) -> (47.9899, 37.6408)
  line L154 (47.9899, 37.6408) -> (47.9899, 37.8171)
  line L155 (47.9899, 37.8171) -> (48.6195, 37.8171)
  line L156 (48.6195, 37.8171) -> (48.6195, 38.217)
  spline S92 degree 2 poles (48.6195, 38.217) (48.5831, 38.2121) (48.5126, 38.2085) (48.4834, 38.2085) knots 0 0 0 1 2 2 2
  spline S93 degree 2 poles (48.4834, 38.2085) (48.3679, 38.2085) (48.2087, 38.2462) (48.1357, 38.3021) knots 0 0 0 1 2 2 2
  spline S94 degree 2 poles (48.1357, 38.3021) (48.0616, 38.358) (47.9814, 38.5282) (47.9814, 38.6643) knots 0 0 0 1 2 2 2
  line L157 (46.6345, 37.6408) -> (47.1511, 39.1408)
  line L158 (47.1511, 39.1408) -> (47.3663, 39.1408)
  line L159 (47.3663, 39.1408) -> (47.8829, 37.6408)
  line L160 (47.8829, 37.6408) -> (47.669, 37.6408)
  line L161 (47.669, 37.6408) -> (47.2532, 38.8868)
  line L162 (47.2532, 38.8868) -> (46.8375, 37.6408)
  line L163 (46.8375, 37.6408) -> (46.6345, 37.6408)
  spline S95 degree 2 poles (48.2196, 41.67) (48.3788, 41.67) (48.6426, 41.5727) (48.7374, 41.4743) knots 0 0 0 1 2 2 2
  spline S96 degree 2 poles (48.7374, 41.4743) (48.8323, 41.3746) (48.9331, 41.0804) (48.9331, 40.8896) knots 0 0 0 1 2 2 2
  spline S97 degree 2 poles (48.9331, 40.8896) (48.9331, 40.7085) (48.831, 40.4216) (48.7362, 40.3195) knots 0 0 0 1 2 2 2
  spline S98 degree 2 poles (48.7362, 40.3195) (48.6451, 40.221) (48.3776, 40.1141) (48.2184, 40.1141) knots 0 0 0 1 2 2 2
  spline S99 degree 2 poles (48.2184, 40.1141) (48.1418, 40.1141) (48.0032, 40.1359) (47.94, 40.1554) knots 0 0 0 1 2 2 2
  spline S100 degree 2 poles (47.94, 40.1554) (47.889, 40.17) (47.765, 40.2235) (47.7273, 40.2429) knots 0 0 0 1 2 2 2
  line L164 (47.7273, 40.2429) -> (47.7273, 40.4836)
  line L165 (47.7273, 40.4836) -> (47.7443, 40.4836)
  spline S101 degree 2 poles (47.7443, 40.4836) (47.782, 40.4508) (47.861, 40.3912) (47.934, 40.3572) knots 0 0 0 1 2 2 2
  spline S102 degree 2 poles (47.934, 40.3572) (47.9947, 40.3268) (48.1515, 40.2867) (48.2415, 40.2867) knots 0 0 0 1 2 2 2
  spline S103 degree 2 poles (48.2415, 40.2867) (48.4579, 40.2867) (48.7253, 40.6124) (48.7253, 40.8835) knots 0 0 0 1 2 2 2
  spline S104 degree 2 poles (48.7253, 40.8835) (48.7253, 41.0342) (48.6548, 41.2603) (48.5879, 41.3381) knots 0 0 0 1 2 2 2
  spline S105 degree 2 poles (48.5879, 41.3381) (48.5235, 41.4159) (48.3412, 41.4974) (48.2269, 41.4974) knots 0 0 0 1 2 2 2
  spline S106 degree 2 poles (48.2269, 41.4974) (48.143, 41.4974) (47.9753, 41.4731) (47.9182, 41.4487) knots 0 0 0 1 2 2 2
  line L166 (47.9182, 41.4487) -> (47.9182, 41.061)
  line L167 (47.9182, 41.061) -> (48.2658, 41.061)
  line L168 (48.2658, 41.061) -> (48.2658, 40.8859)
  line L169 (48.2658, 40.8859) -> (47.7212, 40.8859)
  line L170 (47.7212, 40.8859) -> (47.7212, 41.5411)
  spline S107 degree 2 poles (47.7212, 41.5411) (47.7589, 41.5581) (47.8878, 41.6104) (47.9425, 41.6262) knots 0 0 0 1 2 2 2
  spline S108 degree 2 poles (47.9425, 41.6262) (48.0166, 41.6481) (48.1357, 41.67) (48.2196, 41.67) knots 0 0 0 1 2 2 2
  line L171 (46.3975, 41.6408) -> (46.6212, 41.6408)
  line L172 (46.6212, 41.6408) -> (47.2848, 40.3474)
  line L173 (47.2848, 40.3474) -> (47.2848, 41.6408)
  line L174 (47.2848, 41.6408) -> (47.4708, 41.6408)
  line L175 (47.4708, 41.6408) -> (47.4708, 40.1408)
  line L176 (47.4708, 40.1408) -> (47.1876, 40.1408)
  line L177 (47.1876, 40.1408) -> (46.5835, 41.3284)
  line L178 (46.5835, 41.3284) -> (46.5835, 40.1408)
  line L179 (46.5835, 40.1408) -> (46.3975, 40.1408)
  line L180 (46.3975, 40.1408) -> (46.3975, 41.6408)
  spline S109 degree 2 poles (44.9109, 40.892) (44.9109, 41.0974) (45.0774, 41.4281) (45.2172, 41.5205) knots 0 0 0 1 2 2 2
  spline S110 degree 2 poles (45.2172, 41.5205) (45.3314, 41.5922) (45.566, 41.6408) (45.7484, 41.6408) knots 0 0 0 1 2 2 2
  line L181 (45.7484, 41.6408) -> (46.0936, 41.6408)
  line L182 (46.0936, 41.6408) -> (46.0936, 40.1408)
  line L183 (46.0936, 40.1408) -> (45.752, 40.1408)
  spline S111 degree 2 poles (45.752, 40.1408) (45.5405, 40.1408) (45.2998, 40.204) (45.2147, 40.2599) knots 0 0 0 1 2 2 2
  spline S112 degree 2 poles (45.2147, 40.2599) (45.0701, 40.356) (44.9109, 40.6732) (44.9109, 40.892) knots 0 0 0 1 2 2 2
  spline S113 degree 2 poles (45.1187, 40.8896) (45.1187, 40.717) (45.233, 40.4726) (45.346, 40.4034) knots 0 0 0 1 2 2 2
  spline S114 degree 2 poles (45.346, 40.4034) (45.4263, 40.356) (45.6074, 40.3134) (45.7423, 40.3134) knots 0 0 0 1 2 2 2
  line L184 (45.7423, 40.3134) -> (45.8942, 40.3134)
  line L185 (45.8942, 40.3134) -> (45.8942, 41.4682)
  line L186 (45.8942, 41.4682) -> (45.7423, 41.4682)
  spline S115 degree 2 poles (45.7423, 41.4682) (45.6098, 41.4682) (45.4092, 41.4256) (45.3278, 41.3685) knots 0 0 0 1 2 2 2
  spline S116 degree 2 poles (45.3278, 41.3685) (45.2233, 41.298) (45.1187, 41.0646) (45.1187, 40.8896) knots 0 0 0 1 2 2 2
  spline S117 degree 2 poles (48.2196, 44.17) (48.3788, 44.17) (48.6426, 44.0727) (48.7374, 43.9743) knots 0 0 0 1 2 2 2
  spline S118 degree 2 poles (48.7374, 43.9743) (48.8323, 43.8746) (48.9331, 43.5804) (48.9331, 43.3896) knots 0 0 0 1 2 2 2
  spline S119 degree 2 poles (48.9331, 43.3896) (48.9331, 43.2085) (48.831, 42.9216) (48.7362, 42.8195) knots 0 0 0 1 2 2 2
  spline S120 degree 2 poles (48.7362, 42.8195) (48.6451, 42.721) (48.3776, 42.6141) (48.2184, 42.6141) knots 0 0 0 1 2 2 2
  spline S121 degree 2 poles (48.2184, 42.6141) (48.1418, 42.6141) (48.0032, 42.6359) (47.94, 42.6554) knots 0 0 0 1 2 2 2
  spline S122 degree 2 poles (47.94, 42.6554) (47.889, 42.67) (47.765, 42.7235) (47.7273, 42.7429) knots 0 0 0 1 2 2 2
  line L187 (47.7273, 42.7429) -> (47.7273, 42.9836)
  line L188 (47.7273, 42.9836) -> (47.7443, 42.9836)
  spline S123 degree 2 poles (47.7443, 42.9836) (47.782, 42.9508) (47.861, 42.8912) (47.934, 42.8572) knots 0 0 0 1 2 2 2
  spline S124 degree 2 poles (47.934, 42.8572) (47.9947, 42.8268) (48.1515, 42.7867) (48.2415, 42.7867) knots 0 0 0 1 2 2 2
  spline S125 degree 2 poles (48.2415, 42.7867) (48.4579, 42.7867) (48.7253, 43.1124) (48.7253, 43.3835) knots 0 0 0 1 2 2 2
  spline S126 degree 2 poles (48.7253, 43.3835) (48.7253, 43.5342) (48.6548, 43.7603) (48.5879, 43.8381) knots 0 0 0 1 2 2 2
  spline S127 degree 2 poles (48.5879, 43.8381) (48.5235, 43.9159) (48.3412, 43.9974) (48.2269, 43.9974) knots 0 0 0 1 2 2 2
  spline S128 degree 2 poles (48.2269, 43.9974) (48.143, 43.9974) (47.9753, 43.9731) (47.9182, 43.9487) knots 0 0 0 1 2 2 2
  line L189 (47.9182, 43.9487) -> (47.9182, 43.561)
  line L190 (47.9182, 43.561) -> (48.2658, 43.561)
  line L191 (48.2658, 43.561) -> (48.2658, 43.3859)
  line L192 (48.2658, 43.3859) -> (47.7212, 43.3859)
  line L193 (47.7212, 43.3859) -> (47.7212, 44.0411)
  spline S129 degree 2 poles (47.7212, 44.0411) (47.7589, 44.0581) (47.8878, 44.1104) (47.9425, 44.1262) knots 0 0 0 1 2 2 2
  spline S130 degree 2 poles (47.9425, 44.1262) (48.0166, 44.1481) (48.1357, 44.17) (48.2196, 44.17) knots 0 0 0 1 2 2 2
  line L194 (46.3975, 44.1408) -> (46.6212, 44.1408)
  line L195 (46.6212, 44.1408) -> (47.2848, 42.8474)
  line L196 (47.2848, 42.8474) -> (47.2848, 44.1408)
  line L197 (47.2848, 44.1408) -> (47.4708, 44.1408)
  line L198 (47.4708, 44.1408) -> (47.4708, 42.6408)
  line L199 (47.4708, 42.6408) -> (47.1876, 42.6408)
  line L200 (47.1876, 42.6408) -> (46.5835, 43.8284)
  line L201 (46.5835, 43.8284) -> (46.5835, 42.6408)
  line L202 (46.5835, 42.6408) -> (46.3975, 42.6408)
  line L203 (46.3975, 42.6408) -> (46.3975, 44.1408)
  spline S131 degree 2 poles (44.9109, 43.392) (44.9109, 43.5974) (45.0774, 43.9281) (45.2172, 44.0205) knots 0 0 0 1 2 2 2
  spline S132 degree 2 poles (45.2172, 44.0205) (45.3314, 44.0922) (45.566, 44.1408) (45.7484, 44.1408) knots 0 0 0 1 2 2 2
  line L204 (45.7484, 44.1408) -> (46.0936, 44.1408)
  line L205 (46.0936, 44.1408) -> (46.0936, 42.6408)
  line L206 (46.0936, 42.6408) -> (45.752, 42.6408)
  spline S133 degree 2 poles (45.752, 42.6408) (45.5405, 42.6408) (45.2998, 42.704) (45.2147, 42.7599) knots 0 0 0 1 2 2 2
  spline S134 degree 2 poles (45.2147, 42.7599) (45.0701, 42.856) (44.9109, 43.1732) (44.9109, 43.392) knots 0 0 0 1 2 2 2
  spline S135 degree 2 poles (45.1187, 43.3896) (45.1187, 43.217) (45.233, 42.9726) (45.346, 42.9034) knots 0 0 0 1 2 2 2
  spline S136 degree 2 poles (45.346, 42.9034) (45.4263, 42.856) (45.6074, 42.8134) (45.7423, 42.8134) knots 0 0 0 1 2 2 2
  line L207 (45.7423, 42.8134) -> (45.8942, 42.8134)
  line L208 (45.8942, 42.8134) -> (45.8942, 43.9682)
  line L209 (45.8942, 43.9682) -> (45.7423, 43.9682)
  spline S137 degree 2 poles (45.7423, 43.9682) (45.6098, 43.9682) (45.4092, 43.9256) (45.3278, 43.8685) knots 0 0 0 1 2 2 2
  spline S138 degree 2 poles (45.3278, 43.8685) (45.2233, 43.798) (45.1187, 43.5646) (45.1187, 43.3896) knots 0 0 0 1 2 2 2
  line L210 (47.7601, 45.1408) -> (48.2767, 46.6408)
  line L211 (48.2767, 46.6408) -> (48.4919, 46.6408)
  line L212 (48.4919, 46.6408) -> (49.0085, 45.1408)
  line L213 (49.0085, 45.1408) -> (48.7946, 45.1408)
  line L214 (48.7946, 45.1408) -> (48.3788, 46.3868)
  line L215 (48.3788, 46.3868) -> (47.9631, 45.1408)
  line L216 (47.9631, 45.1408) -> (47.7601, 45.1408)
  line L217 (47.438, 46.6408) -> (47.6276, 46.6408)
  line L218 (47.6276, 46.6408) -> (47.6276, 45.5152)
  line L219 (47.6276, 45.5152) -> (47.438, 45.5152)
  line L220 (47.438, 45.5152) -> (47.438, 46.6408)
  line L221 (47.4246, 45.328) -> (47.6398, 45.328)
  line L222 (47.6398, 45.328) -> (47.6398, 45.1311)
  line L223 (47.6398, 45.1311) -> (47.4246, 45.1311)
  line L224 (47.4246, 45.1311) -> (47.4246, 45.328)
  line L225 (46.2759, 46.6408) -> (46.4656, 46.6408)
  line L226 (46.4656, 46.6408) -> (46.4656, 45.999)
  spline S139 degree 2 poles (46.4656, 45.999) (46.4656, 45.9212) (46.4801, 45.7875) (46.502, 45.7474) knots 0 0 0 1 2 2 2
  spline S140 degree 2 poles (46.502, 45.7474) (46.5251, 45.7048) (46.6078, 45.6635) (46.6783, 45.6635) knots 0 0 0 1 2 2 2
  spline S141 degree 2 poles (46.6783, 45.6635) (46.7488, 45.6635) (46.8983, 45.7389) (46.97, 45.7996) knots 0 0 0 1 2 2 2
  line L227 (46.97, 45.7996) -> (46.97, 46.6408)
  line L228 (46.97, 46.6408) -> (47.1596, 46.6408)
  line L229 (47.1596, 46.6408) -> (47.1596, 45.5152)
  line L230 (47.1596, 45.5152) -> (46.97, 45.5152)
  line L231 (46.97, 45.5152) -> (46.97, 45.6404)
  spline S142 degree 2 poles (46.97, 45.6404) (46.8849, 45.5638) (46.7208, 45.4836) (46.6284, 45.4836) knots 0 0 0 1 2 2 2
  spline S143 degree 2 poles (46.6284, 45.4836) (46.4631, 45.4836) (46.2759, 45.7024) (46.2759, 45.9103) knots 0 0 0 1 2 2 2
  line L232 (46.2759, 45.9103) -> (46.2759, 46.6408)
  line L233 (49.0097, 50.9994) -> (48.5041, 49.4994)
  line L234 (48.5041, 49.4994) -> (48.2585, 49.4994)
  line L235 (48.2585, 49.4994) -> (47.7528, 50.9994)
  line L236 (47.7528, 50.9994) -> (47.9631, 50.9994)
  line L237 (47.9631, 50.9994) -> (48.0993, 50.58)
  line L238 (48.0993, 50.58) -> (48.6718, 50.58)
  line L239 (48.6718, 50.58) -> (48.8079, 50.9994)
  line L240 (48.8079, 50.9994) -> (49.0097, 50.9994)
  line L241 (48.154, 50.4098) -> (48.3861, 49.7036)
  line L242 (48.3861, 49.7036) -> (48.6171, 50.4098)
  line L243 (48.6171, 50.4098) -> (48.154, 50.4098)
  spline S144 degree 2 poles (46.7196, 50.2494) (46.7196, 50.653) (46.9542, 51.031) (47.1985, 51.031) knots 0 0 0 1 2 2 2
  spline S145 degree 2 poles (47.1985, 51.031) (47.4465, 51.031) (47.6787, 50.6457) (47.6787, 50.2506) knots 0 0 0 1 2 2 2
  spline S146 degree 2 poles (47.6787, 50.2506) (47.6787, 49.8446) (47.4441, 49.469) (47.1985, 49.469) knots 0 0 0 1 2 2 2
  spline S147 degree 2 poles (47.1985, 49.469) (46.9518, 49.469) (46.7196, 49.858) (46.7196, 50.2494) knots 0 0 0 1 2 2 2
  spline S148 degree 2 poles (46.9773, 50.7064) (46.9481, 50.6323) (46.9238, 50.4038) (46.9238, 50.2494) knots 0 0 0 1 2 2 2
  spline S149 degree 2 poles (46.9238, 50.2494) (46.9238, 50.095) (46.9481, 49.8677) (46.9785, 49.7911) knots 0 0 0 1 2 2 2
  spline S150 degree 2 poles (46.9785, 49.7911) (47.0089, 49.7145) (47.1147, 49.6355) (47.1985, 49.6355) knots 0 0 0 1 2 2 2
  spline S151 degree 2 poles (47.1985, 49.6355) (47.2824, 49.6355) (47.3906, 49.7145) (47.4222, 49.7936) knots 0 0 0 1 2 2 2
  spline S152 degree 2 poles (47.4222, 49.7936) (47.4526, 49.8701) (47.4745, 50.1035) (47.4745, 50.2506) knots 0 0 0 1 2 2 2
  spline S153 degree 2 poles (47.4745, 50.2506) (47.4745, 50.4086) (47.455, 50.6201) (47.4234, 50.7028) knots 0 0 0 1 2 2 2
  spline S154 degree 2 poles (47.4234, 50.7028) (47.3942, 50.7806) (47.2861, 50.8645) (47.1985, 50.8645) knots 0 0 0 1 2 2 2
  spline S155 degree 2 poles (47.1985, 50.8645) (47.1159, 50.8645) (47.0077, 50.7855) (46.9773, 50.7064) knots 0 0 0 1 2 2 2
  line L244 (49.0097, 53.4994) -> (48.5041, 51.9994)
  line L245 (48.5041, 51.9994) -> (48.2585, 51.9994)
  line L246 (48.2585, 51.9994) -> (47.7528, 53.4994)
  line L247 (47.7528, 53.4994) -> (47.9631, 53.4994)
  line L248 (47.9631, 53.4994) -> (48.0993, 53.08)
  line L249 (48.0993, 53.08) -> (48.6718, 53.08)
  line L250 (48.6718, 53.08) -> (48.8079, 53.4994)
  line L251 (48.8079, 53.4994) -> (49.0097, 53.4994)
  line L252 (48.154, 52.9098) -> (48.3861, 52.2036)
  line L253 (48.3861, 52.2036) -> (48.6171, 52.9098)
  line L254 (48.6171, 52.9098) -> (48.154, 52.9098)
  line L255 (46.8035, 53.4994) -> (47.5353, 53.4994)
  line L256 (47.5353, 53.4994) -> (47.5353, 53.3462)
  line L257 (47.5353, 53.3462) -> (47.263, 53.3462)
  line L258 (47.263, 53.3462) -> (47.263, 52.341)
  line L259 (47.263, 52.341) -> (47.5353, 52.341)
  line L260 (47.5353, 52.341) -> (47.5353, 52.2036)
  spline S156 degree 2 poles (47.5353, 52.2036) (47.3809, 52.2036) (47.235, 52.1161) (47.2253, 51.9945) knots 0 0 0 1 2 2 2
  line L261 (47.2253, 51.9945) -> (47.0697, 51.9945)
  line L262 (47.0697, 51.9945) -> (47.0697, 53.3462)
  line L263 (47.0697, 53.3462) -> (46.8035, 53.3462)
  line L264 (46.8035, 53.3462) -> (46.8035, 53.4994)
  line L265 (49.0097, 55.9994) -> (48.5041, 54.4994)
  line L266 (48.5041, 54.4994) -> (48.2585, 54.4994)
  line L267 (48.2585, 54.4994) -> (47.7528, 55.9994)
  line L268 (47.7528, 55.9994) -> (47.9631, 55.9994)
  line L269 (47.9631, 55.9994) -> (48.0993, 55.58)
  line L270 (48.0993, 55.58) -> (48.6718, 55.58)
  line L271 (48.6718, 55.58) -> (48.8079, 55.9994)
  line L272 (48.8079, 55.9994) -> (49.0097, 55.9994)
  line L273 (48.154, 55.4098) -> (48.3861, 54.7036)
  line L274 (48.3861, 54.7036) -> (48.6171, 55.4098)
  line L275 (48.6171, 55.4098) -> (48.154, 55.4098)
  line L276 (46.7281, 55.9994) -> (47.6532, 55.9994)
  line L277 (47.6532, 55.9994) -> (47.6532, 55.7867)
  spline S157 degree 2 poles (47.6532, 55.7867) (47.5535, 55.6931) (47.376, 55.5192) (47.2909, 55.4256) knots 0 0 0 1 2 2 2
  spline S158 degree 2 poles (47.2909, 55.4256) (47.1195, 55.2372) (46.9943, 55.0111) (46.9943, 54.8908) knots 0 0 0 1 2 2 2
  spline S159 degree 2 poles (46.9943, 54.8908) (46.9943, 54.8276) (47.0332, 54.7328) (47.0685, 54.7024) knots 0 0 0 1 2 2 2
  spline S160 degree 2 poles (47.0685, 54.7024) (47.1037, 54.672) (47.1961, 54.6416) (47.252, 54.6416) knots 0 0 0 1 2 2 2
  spline S161 degree 2 poles (47.252, 54.6416) (47.3055, 54.6416) (47.4149, 54.6684) (47.4647, 54.689) knots 0 0 0 1 2 2 2
  spline S162 degree 2 poles (47.4647, 54.689) (47.5073, 54.706) (47.5863, 54.7547) (47.6106, 54.7717) knots 0 0 0 1 2 2 2
  line L278 (47.6106, 54.7717) -> (47.6216, 54.7717)
  line L279 (47.6216, 54.7717) -> (47.6216, 54.5577)
  spline S163 degree 2 poles (47.6216, 54.5577) (47.5596, 54.5274) (47.3371, 54.4678) (47.2374, 54.4678) knots 0 0 0 1 2 2 2
  spline S164 degree 2 poles (47.2374, 54.4678) (47.0271, 54.4678) (46.7901, 54.6902) (46.7901, 54.8799) knots 0 0 0 1 2 2 2
  spline S165 degree 2 poles (46.7901, 54.8799) (46.7901, 54.9686) (46.8314, 55.1169) (46.8679, 55.1801) knots 0 0 0 1 2 2 2
  spline S166 degree 2 poles (46.8679, 55.1801) (46.9044, 55.2457) (47.0101, 55.3746) (47.0685, 55.4366) knots 0 0 0 1 2 2 2
  spline S167 degree 2 poles (47.0685, 55.4366) (47.1633, 55.5399) (47.3955, 55.7611) (47.4647, 55.8256) knots 0 0 0 1 2 2 2
  line L280 (47.4647, 55.8256) -> (46.7281, 55.8256)
  line L281 (46.7281, 55.8256) -> (46.7281, 55.9994)
  line L282 (49.0097, 58.4994) -> (48.5041, 56.9994)
  line L283 (48.5041, 56.9994) -> (48.2585, 56.9994)
  line L284 (48.2585, 56.9994) -> (47.7528, 58.4994)
  line L285 (47.7528, 58.4994) -> (47.9631, 58.4994)
  line L286 (47.9631, 58.4994) -> (48.0993, 58.08)
  line L287 (48.0993, 58.08) -> (48.6718, 58.08)
  line L288 (48.6718, 58.08) -> (48.8079, 58.4994)
  line L289 (48.8079, 58.4994) -> (49.0097, 58.4994)
  line L290 (48.154, 57.9098) -> (48.3861, 57.2036)
  line L291 (48.3861, 57.2036) -> (48.6171, 57.9098)
  line L292 (48.6171, 57.9098) -> (48.154, 57.9098)